Autodesk Fusion 360 part; units mm, degrees
note: some values were not read from the file. Chosen so that the rebuilt part matches the saved one: which bodies a step acts on; which sketch regions a step uses.
(part 5 of 6)
  line L2431 (-63.4833, -19.2831) -> (-62.2333, -17.118)
  line L2432 (-58.4101, -17.868) -> (-60.9101, -17.868)
  line L2433 (-67.2824, -20.0331) -> (-68.5324, -17.868)
  line L2434 (-88.7768, -22.1981) -> (-87.5268, -20.0331)
  line L2435 (-57.1601, -20.0331) -> (-58.4101, -17.868)
  line L2436 (-81.1546, -22.1981) -> (-78.6546, -22.1981)
  line L2437 (-98.899, -16.5315) -> (-97.649, -14.3664)
  line L2438 (-53.3611, -19.2831) -> (-52.1111, -17.118)
  line L2439 (-92.6, -17.118) -> (-93.85, -14.9529)
  line L2440 (-88.7768, -17.868) -> (-91.2768, -17.868)
  line L2441 (-91.2768, -17.868) -> (-92.5268, -20.0331)
  line L2442 (-62.2333, -17.118) -> (-63.4833, -14.9529)
  line L2443 (-7.799, -17.868) -> (-10.299, -17.868)
  line L2444 (-92.5268, -20.0331) -> (-91.2768, -22.1981)
  line L2445 (-78.6546, -22.1981) -> (-77.4046, -20.0331)
  line L2446 (-93.85, -14.9529) -> (-96.35, -14.9529)
  line L2447 (-96.35, -14.9529) -> (-97.6, -17.118)
  line L2448 (-82.4778, -17.118) -> (-83.7278, -14.9529)
  line L2449 (-73.6056, -19.2831) -> (-72.3556, -17.118)
  line L2450 (-6.5, -17.118) -> (-5.25, -19.2831)
  line L2451 (-50.7879, -22.1981) -> (-48.2879, -22.1981)
  line L2452 (-72.2824, -20.0331) -> (-71.0324, -22.1981)
  line L2453 (-101.399, -17.868) -> (-102.649, -20.0331)
  line L2454 (-58.4101, -22.1981) -> (-57.1601, -20.0331)
  line L2455 (-62.1601, -20.0331) -> (-60.9101, -22.1981)
  line L2456 (-47.0379, -20.0331) -> (-48.2879, -17.868)
  line L2457 (-98.899, -22.1981) -> (-97.649, -20.0331)
  line L2458 (-82.4046, -20.0331) -> (-81.1546, -22.1981)
  line L2459 (-5.25, -19.2831) -> (-2.75, -19.2831)
  line L2460 (-86.2278, -19.2831) -> (-83.7278, -19.2831)
  line L2461 (-55.8611, -14.9529) -> (-57.1111, -17.118)
  line L2462 (-55.8611, -19.2831) -> (-53.3611, -19.2831)
  line L2463 (-57.1111, -17.118) -> (-55.8611, -19.2831)
  line L2464 (-81.1546, -17.868) -> (-82.4046, -20.0331)
  line L2465 (-36.9157, -25.6997) -> (-38.1657, -23.5347)
  line L2466 (-52.0379, -25.6997) -> (-50.7879, -27.8648)
  line L2467 (-53.3611, -24.9497) -> (-52.1111, -22.7847)
  line L2468 (-50.7879, -27.8648) -> (-48.2879, -27.8648)
  line L2469 (-5.25, -20.6196) -> (-6.5, -22.7847)
  line L2470 (-28.0435, -27.8648) -> (-26.7935, -25.6997)
  line L2471 (-30.5435, -23.5347) -> (-31.7935, -25.6997)
  line L2472 (-38.1657, -23.5347) -> (-40.6657, -23.5347)
  line L2473 (-21.7444, -22.7847) -> (-22.9944, -20.6196)
  line L2474 (-68.5324, -17.868) -> (-71.0324, -17.868)
  line L2475 (-45.7389, -20.6196) -> (-46.9889, -22.7847)
  line L2476 (-71.0324, -17.868) -> (-72.2824, -20.0331)
  line L2477 (-22.9944, -24.9497) -> (-21.7444, -22.7847)
  line L2478 (-43.2389, -24.9497) -> (-41.9889, -22.7847)
  line L2479 (-36.8667, -22.7847) -> (-35.6167, -24.9497)
  line L2480 (-7.799, -27.8648) -> (-6.549, -25.6997)
  line L2481 (-40.6657, -23.5347) -> (-41.9157, -25.6997)
  line L2482 (-35.6167, -24.9497) -> (-33.1167, -24.9497)
  line L2483 (-22.9944, -20.6196) -> (-25.4944, -20.6196)
  line L2484 (-35.6167, -20.6196) -> (-36.8667, -22.7847)
  line L2485 (-48.2879, -22.1981) -> (-47.0379, -20.0331)
  line L2486 (-21.6713, -25.6997) -> (-20.4213, -27.8648)
  line L2487 (-38.1657, -27.8648) -> (-36.9157, -25.6997)
  line L2488 (-93.85, -19.2831) -> (-92.6, -17.118)
  line L2489 (-11.6222, -22.7847) -> (-12.8722, -20.6196)
  line L2490 (-20.4213, -23.5347) -> (-21.6713, -25.6997)
  line L2491 (-96.35, -19.2831) -> (-93.85, -19.2831)
  line L2492 (-5.25, -24.9497) -> (-2.75, -24.9497)
  line L2493 (-97.649, -20.0331) -> (-98.899, -17.868)
  line L2494 (-2.75, -24.9497) -> (-1.5, -22.7847)
  line L2495 (-16.6713, -25.6997) -> (-17.9213, -23.5347)
  line L2496 (-6.549, -25.6997) -> (-7.799, -23.5347)
  line L2497 (-41.9157, -25.6997) -> (-40.6657, -27.8648)
  line L2498 (-17.9213, -23.5347) -> (-20.4213, -23.5347)
  line L2499 (-31.8667, -22.7847) -> (-33.1167, -20.6196)
  line L2500 (-12.8722, -24.9497) -> (-11.6222, -22.7847)
  line L2501 (-17.9213, -27.8648) -> (-16.6713, -25.6997)
  line L2502 (-55.8611, -24.9497) -> (-53.3611, -24.9497)
  line L2503 (-6.5, -22.7847) -> (-5.25, -24.9497)
  line L2504 (-53.3611, -20.6196) -> (-55.8611, -20.6196)
  line L2505 (-33.1167, -24.9497) -> (-31.8667, -22.7847)
  line L2506 (-30.5435, -27.8648) -> (-28.0435, -27.8648)
  line L2507 (-31.7935, -25.6997) -> (-30.5435, -27.8648)
  line L2508 (-2.75, -20.6196) -> (-5.25, -20.6196)
  line L2509 (-45.7389, -24.9497) -> (-43.2389, -24.9497)
  line L2510 (-26.7935, -25.6997) -> (-28.0435, -23.5347)
  line L2511 (-11.549, -25.6997) -> (-10.299, -27.8648)
  line L2512 (-55.8611, -20.6196) -> (-57.1111, -22.7847)
  line L2513 (-41.9889, -22.7847) -> (-43.2389, -20.6196)
  line L2514 (-57.1111, -22.7847) -> (-55.8611, -24.9497)
  line L2515 (-77.3556, -17.118) -> (-76.1056, -19.2831)
  line L2516 (-1.5, -22.7847) -> (-2.75, -20.6196)
  line L2517 (-47.0379, -25.6997) -> (-48.2879, -23.5347)
  line L2518 (-12.8722, -20.6196) -> (-15.3722, -20.6196)
  line L2519 (-40.6657, -27.8648) -> (-38.1657, -27.8648)
  line L2520 (-20.4213, -27.8648) -> (-17.9213, -27.8648)
  line L2521 (-71.0324, -22.1981) -> (-68.5324, -22.1981)
  line L2522 (-87.4778, -17.118) -> (-86.2278, -19.2831)
  line L2523 (-48.2879, -23.5347) -> (-50.7879, -23.5347)
  line L2524 (-26.7444, -22.7847) -> (-25.4944, -24.9497)
  line L2525 (-65.9833, -19.2831) -> (-63.4833, -19.2831)
  line L2526 (-28.0435, -23.5347) -> (-30.5435, -23.5347)
  line L2527 (-43.2389, -20.6196) -> (-45.7389, -20.6196)
  line L2528 (-48.2879, -27.8648) -> (-47.0379, -25.6997)
  line L2529 (-2.75, -26.2863) -> (-5.25, -26.2863)
  line L2530 (-71.0324, -23.5347) -> (-72.2824, -25.6997)
  line L2531 (-68.5324, -27.8648) -> (-67.2824, -25.6997)
  line L2532 (-11.549, -31.3664) -> (-10.299, -33.5315)
  line L2533 (-91.2768, -27.8648) -> (-88.7768, -27.8648)
  line L2534 (-81.1546, -27.8648) -> (-78.6546, -27.8648)
  line L2535 (-93.85, -24.9497) -> (-92.6, -22.7847)
  line L2536 (-10.299, -23.5347) -> (-11.549, -25.6997)
  line L2537 (-15.3722, -24.9497) -> (-12.8722, -24.9497)
  line L2538 (-78.6546, -23.5347) -> (-81.1546, -23.5347)
  line L2539 (-60.9101, -23.5347) -> (-62.1601, -25.6997)
  line L2540 (-81.1546, -23.5347) -> (-82.4046, -25.6997)
  line L2541 (-65.9833, -20.6196) -> (-67.2333, -22.7847)
  line L2542 (-33.1167, -20.6196) -> (-35.6167, -20.6196)
  line L2543 (-58.4101, -23.5347) -> (-60.9101, -23.5347)
  line L2544 (-76.1056, -20.6196) -> (-77.3556, -22.7847)
  line L2545 (-25.4944, -24.9497) -> (-22.9944, -24.9497)
  line L2546 (-86.2278, -24.9497) -> (-83.7278, -24.9497)
  line L2547 (-97.6, -22.7847) -> (-96.35, -24.9497)
  line L2548 (-6.5, -28.4513) -> (-5.25, -30.6164)
  line L2549 (-63.4833, -20.6196) -> (-65.9833, -20.6196)
  line L2550 (-65.9833, -24.9497) -> (-63.4833, -24.9497)
  line L2551 (-88.7768, -27.8648) -> (-87.5268, -25.6997)
  line L2552 (-67.2824, -25.6997) -> (-68.5324, -23.5347)
  line L2553 (-2.75, -30.6164) -> (-1.5, -28.4513)
  line L2554 (-93.85, -20.6196) -> (-96.35, -20.6196)
  line L2555 (-98.899, -23.5347) -> (-101.399, -23.5347)
  line L2556 (-62.2333, -22.7847) -> (-63.4833, -20.6196)
  line L2557 (-92.6, -22.7847) -> (-93.85, -20.6196)
  line L2558 (-76.1056, -24.9497) -> (-73.6056, -24.9497)
  line L2559 (-96.35, -20.6196) -> (-97.6, -22.7847)
  line L2560 (-97.649, -25.6997) -> (-98.899, -23.5347)
  line L2561 (-7.799, -29.2013) -> (-10.299, -29.2013)
  line L2562 (-83.7278, -20.6196) -> (-86.2278, -20.6196)
  line L2563 (-73.6056, -20.6196) -> (-76.1056, -20.6196)
  line L2564 (-87.5268, -25.6997) -> (-88.7768, -23.5347)
  line L2565 (-83.7278, -24.9497) -> (-82.4778, -22.7847)
  line L2566 (-77.3556, -22.7847) -> (-76.1056, -24.9497)
  line L2567 (-88.7768, -23.5347) -> (-91.2768, -23.5347)
  line L2568 (-7.799, -23.5347) -> (-10.299, -23.5347)
  line L2569 (-15.3722, -20.6196) -> (-16.6222, -22.7847)
  line L2570 (-67.2333, -22.7847) -> (-65.9833, -24.9497)
  line L2571 (-1.5, -28.4513) -> (-2.75, -26.2863)
  line L2572 (-52.1111, -22.7847) -> (-53.3611, -20.6196)
  line L2573 (-25.4944, -20.6196) -> (-26.7444, -22.7847)
  line L2574 (-10.299, -29.2013) -> (-11.549, -31.3664)
  line L2575 (-101.399, -27.8648) -> (-98.899, -27.8648)
  line L2576 (-10.299, -33.5315) -> (-7.799, -33.5315)
  line L2577 (-72.3556, -22.7847) -> (-73.6056, -20.6196)
  line L2578 (-16.6222, -22.7847) -> (-15.3722, -24.9497)
  line L2579 (-92.5268, -25.6997) -> (-91.2768, -27.8648)
  line L2580 (-46.9889, -22.7847) -> (-45.7389, -24.9497)
  line L2581 (-10.299, -27.8648) -> (-7.799, -27.8648)
  line L2582 (-50.7879, -23.5347) -> (-52.0379, -25.6997)
  line L2583 (-58.4101, -27.8648) -> (-57.1601, -25.6997)
  line L2584 (-82.4046, -25.6997) -> (-81.1546, -27.8648)
  line L2585 (-72.2824, -25.6997) -> (-71.0324, -27.8648)
  line L2586 (-5.25, -30.6164) -> (-2.75, -30.6164)
  line L2587 (-87.4778, -22.7847) -> (-86.2278, -24.9497)
  line L2588 (-5.25, -26.2863) -> (-6.5, -28.4513)
  line L2589 (-62.1601, -25.6997) -> (-60.9101, -27.8648)
  line L2590 (-101.399, -23.5347) -> (-102.649, -25.6997)
  line L2591 (-102.649, -25.6997) -> (-101.399, -27.8648)
  line L2592 (-57.1601, -25.6997) -> (-58.4101, -23.5347)
  line L2593 (-30.5435, -33.5315) -> (-28.0435, -33.5315)
  line L2594 (-33.1167, -30.6164) -> (-31.8667, -28.4513)
  line L2595 (-50.7879, -29.2013) -> (-52.0379, -31.3664)
  line L2596 (-43.2389, -30.6164) -> (-41.9889, -28.4513)
  line L2597 (-91.2768, -23.5347) -> (-92.5268, -25.6997)
  line L2598 (-57.1111, -28.4513) -> (-55.8611, -30.6164)
  line L2599 (-20.4213, -33.5315) -> (-17.9213, -33.5315)
  line L2600 (-53.3611, -26.2863) -> (-55.8611, -26.2863)
  line L2601 (-26.7935, -31.3664) -> (-28.0435, -29.2013)
  line L2602 (-50.7879, -33.5315) -> (-48.2879, -33.5315)
  line L2603 (-71.0324, -27.8648) -> (-68.5324, -27.8648)
  line L2604 (-17.9213, -29.2013) -> (-20.4213, -29.2013)
  line L2605 (-26.7444, -28.4513) -> (-25.4944, -30.6164)
  line L2606 (-16.6713, -31.3664) -> (-17.9213, -29.2013)
  line L2607 (-77.4046, -25.6997) -> (-78.6546, -23.5347)
  line L2608 (-41.9157, -31.3664) -> (-40.6657, -33.5315)
  line L2609 (-41.9889, -28.4513) -> (-43.2389, -26.2863)
  line L2610 (-78.6546, -27.8648) -> (-77.4046, -25.6997)
  line L2611 (-86.2278, -20.6196) -> (-87.4778, -22.7847)
  line L2612 (-15.3722, -30.6164) -> (-12.8722, -30.6164)
  line L2613 (-63.4833, -24.9497) -> (-62.2333, -22.7847)
  line L2614 (-53.3611, -30.6164) -> (-52.1111, -28.4513)
  line L2615 (-40.6657, -33.5315) -> (-38.1657, -33.5315)
  line L2616 (-55.8611, -30.6164) -> (-53.3611, -30.6164)
  line L2617 (-16.6222, -28.4513) -> (-15.3722, -30.6164)
  line L2618 (-21.6713, -31.3664) -> (-20.4213, -33.5315)
  line L2619 (-15.3722, -26.2863) -> (-16.6222, -28.4513)
  line L2620 (-43.2389, -26.2863) -> (-45.7389, -26.2863)
  line L2621 (-11.6222, -28.4513) -> (-12.8722, -26.2863)
  line L2622 (-31.7935, -31.3664) -> (-30.5435, -33.5315)
  line L2623 (-28.0435, -29.2013) -> (-30.5435, -29.2013)
  line L2624 (-55.8611, -26.2863) -> (-57.1111, -28.4513)
  line L2625 (-38.1657, -33.5315) -> (-36.9157, -31.3664)
  line L2626 (-28.0435, -33.5315) -> (-26.7935, -31.3664)
  line L2627 (-48.2879, -29.2013) -> (-50.7879, -29.2013)
  line L2628 (-35.6167, -26.2863) -> (-36.8667, -28.4513)
  line L2629 (-98.899, -27.8648) -> (-97.649, -25.6997)
  line L2630 (-25.4944, -26.2863) -> (-26.7444, -28.4513)
  line L2631 (-52.1111, -28.4513) -> (-53.3611, -26.2863)
  line L2632 (-96.35, -24.9497) -> (-93.85, -24.9497)
  line L2633 (-20.4213, -29.2013) -> (-21.6713, -31.3664)
  line L2634 (-12.8722, -26.2863) -> (-15.3722, -26.2863)
  line L2635 (-58.4101, -29.2013) -> (-60.9101, -29.2013)
  line L2636 (-58.4101, -33.5315) -> (-57.1601, -31.3664)
  line L2637 (-52.0379, -31.3664) -> (-50.7879, -33.5315)
  line L2638 (-40.6657, -29.2013) -> (-41.9157, -31.3664)
  line L2639 (-82.4778, -22.7847) -> (-83.7278, -20.6196)
  line L2640 (-31.8667, -28.4513) -> (-33.1167, -26.2863)
  line L2641 (-47.0379, -31.3664) -> (-48.2879, -29.2013)
  line L2642 (-21.7444, -28.4513) -> (-22.9944, -26.2863)
  line L2643 (-60.9101, -27.8648) -> (-58.4101, -27.8648)
  line L2644 (-38.1657, -29.2013) -> (-40.6657, -29.2013)
  line L2645 (-48.2879, -33.5315) -> (-47.0379, -31.3664)
  line L2646 (-36.9157, -31.3664) -> (-38.1657, -29.2013)
  line L2647 (-46.9889, -28.4513) -> (-45.7389, -30.6164)
  line L2648 (-6.549, -31.3664) -> (-7.799, -29.2013)
  line L2649 (-33.1167, -26.2863) -> (-35.6167, -26.2863)
  line L2650 (-45.7389, -26.2863) -> (-46.9889, -28.4513)
  line L2651 (-73.6056, -24.9497) -> (-72.3556, -22.7847)
  line L2652 (-36.8667, -28.4513) -> (-35.6167, -30.6164)
  line L2653 (-17.9213, -33.5315) -> (-16.6713, -31.3664)
  line L2654 (-62.1601, -31.3664) -> (-60.9101, -33.5315)
  line L2655 (-60.9101, -29.2013) -> (-62.1601, -31.3664)
  line L2656 (-68.5324, -23.5347) -> (-71.0324, -23.5347)
  line L2657 (-2.75, -36.2831) -> (-1.5, -34.118)
  line L2658 (-7.799, -34.868) -> (-10.299, -34.868)
  line L2659 (-11.6222, -34.118) -> (-12.8722, -31.9529)
  line L2660 (-83.7278, -26.2863) -> (-86.2278, -26.2863)
  line L2661 (-30.5435, -29.2013) -> (-31.7935, -31.3664)
  line L2662 (-98.899, -33.5315) -> (-97.649, -31.3664)
  line L2663 (-1.5, -34.118) -> (-2.75, -31.9529)
  line L2664 (-81.1546, -29.2013) -> (-82.4046, -31.3664)
  line L2665 (-35.6167, -30.6164) -> (-33.1167, -30.6164)
  line L2666 (-63.4833, -30.6164) -> (-62.2333, -28.4513)
  line L2667 (-67.2824, -31.3664) -> (-68.5324, -29.2013)
  line L2668 (-45.7389, -30.6164) -> (-43.2389, -30.6164)
  line L2669 (-78.6546, -29.2013) -> (-81.1546, -29.2013)
  line L2670 (-97.6, -28.4513) -> (-96.35, -30.6164)
  line L2671 (-25.4944, -30.6164) -> (-22.9944, -30.6164)
  line L2672 (-12.8722, -31.9529) -> (-15.3722, -31.9529)
  line L2673 (-93.85, -26.2863) -> (-96.35, -26.2863)
  line L2674 (-63.4833, -26.2863) -> (-65.9833, -26.2863)
  line L2675 (-87.5268, -31.3664) -> (-88.7768, -29.2013)
  line L2676 (-7.799, -33.5315) -> (-6.549, -31.3664)
  line L2677 (-91.2768, -29.2013) -> (-92.5268, -31.3664)
  line L2678 (-73.6056, -26.2863) -> (-76.1056, -26.2863)
  line L2679 (-102.649, -31.3664) -> (-101.399, -33.5315)
  line L2680 (-7.799, -39.1981) -> (-6.549, -37.0331)
  line L2681 (-11.549, -37.0331) -> (-10.299, -39.1981)
  line L2682 (-73.6056, -30.6164) -> (-72.3556, -28.4513)
  line L2683 (-57.1601, -31.3664) -> (-58.4101, -29.2013)
  line L2684 (-88.7768, -29.2013) -> (-91.2768, -29.2013)
  line L2685 (-22.9944, -30.6164) -> (-21.7444, -28.4513)
  line L2686 (-86.2278, -26.2863) -> (-87.4778, -28.4513)
  line L2687 (-101.399, -33.5315) -> (-98.899, -33.5315)
  line L2688 (-82.4046, -31.3664) -> (-81.1546, -33.5315)
  line L2689 (-92.6, -28.4513) -> (-93.85, -26.2863)
  line L2690 (-67.2333, -28.4513) -> (-65.9833, -30.6164)
  line L2691 (-76.1056, -26.2863) -> (-77.3556, -28.4513)
  line L2692 (-5.25, -31.9529) -> (-6.5, -34.118)
  line L2693 (-72.2824, -31.3664) -> (-71.0324, -33.5315)
  line L2694 (-96.35, -30.6164) -> (-93.85, -30.6164)
  line L2695 (-97.649, -31.3664) -> (-98.899, -29.2013)
  line L2696 (-101.399, -29.2013) -> (-102.649, -31.3664)
  line L2697 (-68.5324, -33.5315) -> (-67.2824, -31.3664)
  line L2698 (-77.3556, -28.4513) -> (-76.1056, -30.6164)
  line L2699 (-91.2768, -33.5315) -> (-88.7768, -33.5315)
  line L2700 (-10.299, -39.1981) -> (-7.799, -39.1981)
  line L2701 (-96.35, -26.2863) -> (-97.6, -28.4513)
  line L2702 (-62.2333, -28.4513) -> (-63.4833, -26.2863)
  line L2703 (-12.8722, -30.6164) -> (-11.6222, -28.4513)
  line L2704 (-60.9101, -33.5315) -> (-58.4101, -33.5315)
  line L2705 (-22.9944, -26.2863) -> (-25.4944, -26.2863)
  line L2706 (-12.8722, -36.2831) -> (-11.6222, -34.118)
  line L2707 (-6.549, -37.0331) -> (-7.799, -34.868)
  line L2708 (-93.85, -30.6164) -> (-92.6, -28.4513)
  line L2709 (-76.1056, -30.6164) -> (-73.6056, -30.6164)
  line L2710 (-68.5324, -29.2013) -> (-71.0324, -29.2013)
  line L2711 (-82.4778, -28.4513) -> (-83.7278, -26.2863)
  line L2712 (-98.899, -29.2013) -> (-101.399, -29.2013)
  line L2713 (-71.0324, -33.5315) -> (-68.5324, -33.5315)
  line L2714 (-72.3556, -28.4513) -> (-73.6056, -26.2863)
  line L2715 (-65.9833, -30.6164) -> (-63.4833, -30.6164)
  line L2716 (-71.0324, -29.2013) -> (-72.2824, -31.3664)
  line L2717 (-10.299, -34.868) -> (-11.549, -37.0331)
  line L2718 (-5.25, -36.2831) -> (-2.75, -36.2831)
  line L2719 (-6.5, -34.118) -> (-5.25, -36.2831)
  line L2720 (-86.2278, -30.6164) -> (-83.7278, -30.6164)
  line L2721 (-30.5435, -34.868) -> (-31.7935, -37.0331)
  line L2722 (-38.1657, -34.868) -> (-40.6657, -34.868)
  line L2723 (-53.3611, -31.9529) -> (-55.8611, -31.9529)
  line L2724 (-58.4101, -39.1981) -> (-57.1601, -37.0331)
  line L2725 (-47.0379, -37.0331) -> (-48.2879, -34.868)
  line L2726 (-31.7935, -37.0331) -> (-30.5435, -39.1981)
  line L2727 (-68.5324, -34.868) -> (-71.0324, -34.868)
  line L2728 (-71.0324, -34.868) -> (-72.2824, -37.0331)
  line L2729 (-46.9889, -34.118) -> (-45.7389, -36.2831)
  line L2730 (-71.0324, -39.1981) -> (-68.5324, -39.1981)
  line L2731 (-17.9213, -34.868) -> (-20.4213, -34.868)
  line L2732 (-41.9889, -34.118) -> (-43.2389, -31.9529)
  line L2733 (-52.0379, -37.0331) -> (-50.7879, -39.1981)
  line L2734 (-17.9213, -39.1981) -> (-16.6713, -37.0331)
  line L2735 (-92.5268, -31.3664) -> (-91.2768, -33.5315)
  line L2736 (-22.9944, -36.2831) -> (-21.7444, -34.118)
  line L2737 (-31.8667, -34.118) -> (-33.1167, -31.9529)
  line L2738 (-41.9157, -37.0331) -> (-40.6657, -39.1981)
  line L2739 (-25.4944, -36.2831) -> (-22.9944, -36.2831)
  line L2740 (-20.4213, -39.1981) -> (-17.9213, -39.1981)
  line L2741 (-65.9833, -36.2831) -> (-63.4833, -36.2831)
  line L2742 (-58.4101, -34.868) -> (-60.9101, -34.868)
  line L2743 (-15.3722, -36.2831) -> (-12.8722, -36.2831)
  line L2744 (-88.7768, -33.5315) -> (-87.5268, -31.3664)
  line L2745 (-30.5435, -39.1981) -> (-28.0435, -39.1981)
  line L2746 (-60.9101, -34.868) -> (-62.1601, -37.0331)
  line L2747 (-25.4944, -31.9529) -> (-26.7444, -34.118)
  line L2748 (-21.6713, -37.0331) -> (-20.4213, -39.1981)
  line L2749 (-40.6657, -39.1981) -> (-38.1657, -39.1981)
  line L2750 (-38.1657, -39.1981) -> (-36.9157, -37.0331)
  line L2751 (-40.6657, -34.868) -> (-41.9157, -37.0331)
  line L2752 (-48.2879, -34.868) -> (-50.7879, -34.868)
  line L2753 (-57.1111, -34.118) -> (-55.8611, -36.2831)
  line L2754 (-52.1111, -34.118) -> (-53.3611, -31.9529)
  line L2755 (-60.9101, -39.1981) -> (-58.4101, -39.1981)
  line L2756 (-28.0435, -39.1981) -> (-26.7935, -37.0331)
  line L2757 (-83.7278, -30.6164) -> (-82.4778, -28.4513)
  line L2758 (-2.75, -31.9529) -> (-5.25, -31.9529)
  line L2759 (-16.6222, -34.118) -> (-15.3722, -36.2831)
  line L2760 (-77.4046, -31.3664) -> (-78.6546, -29.2013)
  line L2761 (-22.9944, -31.9529) -> (-25.4944, -31.9529)
  line L2762 (-26.7444, -34.118) -> (-25.4944, -36.2831)
  line L2763 (-35.6167, -36.2831) -> (-33.1167, -36.2831)
  line L2764 (-65.9833, -31.9529) -> (-67.2333, -34.118)
  line L2765 (-72.2824, -37.0331) -> (-71.0324, -39.1981)
  line L2766 (-16.6713, -37.0331) -> (-17.9213, -34.868)
  line L2767 (-65.9833, -26.2863) -> (-67.2333, -28.4513)
  line L2768 (-62.2333, -34.118) -> (-63.4833, -31.9529)
  line L2769 (-45.7389, -31.9529) -> (-46.9889, -34.118)
  line L2770 (-36.8667, -34.118) -> (-35.6167, -36.2831)
  line L2771 (-62.1601, -37.0331) -> (-60.9101, -39.1981)
  line L2772 (-33.1167, -36.2831) -> (-31.8667, -34.118)
  line L2773 (-50.7879, -34.868) -> (-52.0379, -37.0331)
  line L2774 (-63.4833, -31.9529) -> (-65.9833, -31.9529)
  line L2775 (-43.2389, -31.9529) -> (-45.7389, -31.9529)
  line L2776 (-78.6546, -33.5315) -> (-77.4046, -31.3664)
  line L2777 (-87.4778, -28.4513) -> (-86.2278, -30.6164)
  line L2778 (-63.4833, -36.2831) -> (-62.2333, -34.118)
  line L2779 (-55.8611, -31.9529) -> (-57.1111, -34.118)
  line L2780 (-81.1546, -33.5315) -> (-78.6546, -33.5315)
  line L2781 (-20.4213, -34.868) -> (-21.6713, -37.0331)
  line L2782 (-15.3722, -31.9529) -> (-16.6222, -34.118)
  line L2783 (-33.1167, -31.9529) -> (-35.6167, -31.9529)
  line L2784 (-53.3611, -36.2831) -> (-52.1111, -34.118)
  line L2785 (-5.25, -37.6196) -> (-6.5, -39.7847)
  line L2786 (-21.7444, -34.118) -> (-22.9944, -31.9529)
  line L2787 (-97.6, -34.118) -> (-96.35, -36.2831)
  line L2788 (-36.9157, -37.0331) -> (-38.1657, -34.868)
  line L2789 (-11.549, -42.6997) -> (-10.299, -44.8648)
  line L2790 (-50.7879, -39.1981) -> (-48.2879, -39.1981)
  line L2791 (-15.3722, -41.9497) -> (-12.8722, -41.9497)
  line L2792 (-82.4046, -37.0331) -> (-81.1546, -39.1981)
  line L2793 (-28.0435, -34.868) -> (-30.5435, -34.868)
  line L2794 (-21.6713, -42.6997) -> (-20.4213, -44.8648)
  line L2795 (-15.3722, -37.6196) -> (-16.6222, -39.7847)
  line L2796 (-82.4778, -34.118) -> (-83.7278, -31.9529)
  line L2797 (-92.5268, -37.0331) -> (-91.2768, -39.1981)
  line L2798 (-72.3556, -34.118) -> (-73.6056, -31.9529)
  line L2799 (-11.6222, -39.7847) -> (-12.8722, -37.6196)
  line L2800 (-77.4046, -37.0331) -> (-78.6546, -34.868)
  line L2801 (-26.7935, -37.0331) -> (-28.0435, -34.868)
  line L2802 (-10.299, -44.8648) -> (-7.799, -44.8648)
  line L2803 (-68.5324, -39.1981) -> (-67.2824, -37.0331)
  line L2804 (-86.2278, -36.2831) -> (-83.7278, -36.2831)
  line L2805 (-81.1546, -39.1981) -> (-78.6546, -39.1981)
  line L2806 (-87.5268, -37.0331) -> (-88.7768, -34.868)
  line L2807 (-96.35, -31.9529) -> (-97.6, -34.118)
  line L2808 (-26.7444, -39.7847) -> (-25.4944, -41.9497)
  line L2809 (-102.649, -37.0331) -> (-101.399, -39.1981)
  line L2810 (-12.8722, -37.6196) -> (-15.3722, -37.6196)
  line L2811 (-12.8722, -41.9497) -> (-11.6222, -39.7847)
  line L2812 (-57.1601, -37.0331) -> (-58.4101, -34.868)
  line L2813 (-25.4944, -41.9497) -> (-22.9944, -41.9497)
  line L2814 (-76.1056, -31.9529) -> (-77.3556, -34.118)
  line L2815 (-1.5, -39.7847) -> (-2.75, -37.6196)
  line L2816 (-67.2824, -37.0331) -> (-68.5324, -34.868)
  line L2817 (-91.2768, -39.1981) -> (-88.7768, -39.1981)
  line L2818 (-7.799, -40.5347) -> (-10.299, -40.5347)
  line L2819 (-55.8611, -36.2831) -> (-53.3611, -36.2831)
  line L2820 (-87.4778, -34.118) -> (-86.2278, -36.2831)
  line L2821 (-96.35, -36.2831) -> (-93.85, -36.2831)
  line L2822 (-7.799, -44.8648) -> (-6.549, -42.6997)
  line L2823 (-83.7278, -31.9529) -> (-86.2278, -31.9529)
  line L2824 (-43.2389, -36.2831) -> (-41.9889, -34.118)
  line L2825 (-35.6167, -31.9529) -> (-36.8667, -34.118)
  line L2826 (-97.649, -37.0331) -> (-98.899, -34.868)
  line L2827 (-67.2333, -34.118) -> (-65.9833, -36.2831)
  line L2828 (-98.899, -34.868) -> (-101.399, -34.868)
  line L2829 (-81.1546, -34.868) -> (-82.4046, -37.0331)
  line L2830 (-101.399, -34.868) -> (-102.649, -37.0331)
  line L2831 (-20.4213, -44.8648) -> (-17.9213, -44.8648)
  line L2832 (-48.2879, -39.1981) -> (-47.0379, -37.0331)
  line L2833 (-78.6546, -39.1981) -> (-77.4046, -37.0331)
  line L2834 (-2.75, -41.9497) -> (-1.5, -39.7847)
  line L2835 (-92.6, -34.118) -> (-93.85, -31.9529)
  line L2836 (-93.85, -31.9529) -> (-96.35, -31.9529)
  line L2837 (-78.6546, -34.868) -> (-81.1546, -34.868)
  line L2838 (-45.7389, -36.2831) -> (-43.2389, -36.2831)
  line L2839 (-10.299, -40.5347) -> (-11.549, -42.6997)
  line L2840 (-2.75, -37.6196) -> (-5.25, -37.6196)
  line L2841 (-20.4213, -40.5347) -> (-21.6713, -42.6997)
  line L2842 (-73.6056, -31.9529) -> (-76.1056, -31.9529)
  line L2843 (-6.5, -39.7847) -> (-5.25, -41.9497)
  line L2844 (-73.6056, -36.2831) -> (-72.3556, -34.118)
  line L2845 (-16.6713, -42.6997) -> (-17.9213, -40.5347)
  line L2846 (-76.1056, -36.2831) -> (-73.6056, -36.2831)
  line L2847 (-91.2768, -34.868) -> (-92.5268, -37.0331)
  line L2848 (-17.9213, -40.5347) -> (-20.4213, -40.5347)
  line L2849 (-53.3611, -41.9497) -> (-52.1111, -39.7847)
  line L2850 (-58.4101, -44.8648) -> (-57.1601, -42.6997)
  line L2851 (-31.7935, -42.6997) -> (-30.5435, -44.8648)
  line L2852 (-62.1601, -42.6997) -> (-60.9101, -44.8648)
  line L2853 (-67.2333, -39.7847) -> (-65.9833, -41.9497)
  line L2854 (-22.9944, -37.6196) -> (-25.4944, -37.6196)
  line L2855 (-46.9889, -39.7847) -> (-45.7389, -41.9497)
  line L2856 (-45.7389, -41.9497) -> (-43.2389, -41.9497)
  line L2857 (-40.6657, -44.8648) -> (-38.1657, -44.8648)
  line L2858 (-77.3556, -34.118) -> (-76.1056, -36.2831)
  line L2859 (-30.5435, -40.5347) -> (-31.7935, -42.6997)
  line L2860 (-16.6222, -39.7847) -> (-15.3722, -41.9497)
  line L2861 (-28.0435, -44.8648) -> (-26.7935, -42.6997)
  line L2862 (-28.0435, -40.5347) -> (-30.5435, -40.5347)
  line L2863 (-36.8667, -39.7847) -> (-35.6167, -41.9497)
  line L2864 (-45.7389, -37.6196) -> (-46.9889, -39.7847)
  line L2865 (-26.7935, -42.6997) -> (-28.0435, -40.5347)
  line L2866 (-31.8667, -39.7847) -> (-33.1167, -37.6196)
  line L2867 (-77.3556, -39.7847) -> (-76.1056, -41.9497)
  line L2868 (-41.9157, -42.6997) -> (-40.6657, -44.8648)
  line L2869 (-101.399, -39.1981) -> (-98.899, -39.1981)
  line L2870 (-67.2824, -42.6997) -> (-68.5324, -40.5347)
  line L2871 (-33.1167, -37.6196) -> (-35.6167, -37.6196)
  line L2872 (-98.899, -39.1981) -> (-97.649, -37.0331)
  line L2873 (-73.6056, -41.9497) -> (-72.3556, -39.7847)
  line L2874 (-22.9944, -41.9497) -> (-21.7444, -39.7847)
  line L2875 (-17.9213, -44.8648) -> (-16.6713, -42.6997)
  line L2876 (-86.2278, -31.9529) -> (-87.4778, -34.118)
  line L2877 (-5.25, -41.9497) -> (-2.75, -41.9497)
  line L2878 (-43.2389, -37.6196) -> (-45.7389, -37.6196)
  line L2879 (-60.9101, -40.5347) -> (-62.1601, -42.6997)
  line L2880 (-63.4833, -37.6196) -> (-65.9833, -37.6196)
  line L2881 (-76.1056, -41.9497) -> (-73.6056, -41.9497)
  line L2882 (-76.1056, -37.6196) -> (-77.3556, -39.7847)
  line L2883 (-48.2879, -40.5347) -> (-50.7879, -40.5347)
  line L2884 (-55.8611, -37.6196) -> (-57.1111, -39.7847)
  line L2885 (-52.0379, -42.6997) -> (-50.7879, -44.8648)
  line L2886 (-30.5435, -44.8648) -> (-28.0435, -44.8648)
  line L2887 (-83.7278, -36.2831) -> (-82.4778, -34.118)
  line L2888 (-43.2389, -41.9497) -> (-41.9889, -39.7847)
  line L2889 (-88.7768, -39.1981) -> (-87.5268, -37.0331)
  line L2890 (-73.6056, -37.6196) -> (-76.1056, -37.6196)
  line L2891 (-62.2333, -39.7847) -> (-63.4833, -37.6196)
  line L2892 (-57.1601, -42.6997) -> (-58.4101, -40.5347)
  line L2893 (-40.6657, -40.5347) -> (-41.9157, -42.6997)
  line L2894 (-41.9889, -39.7847) -> (-43.2389, -37.6196)
  line L2895 (-58.4101, -40.5347) -> (-60.9101, -40.5347)
  line L2896 (-47.0379, -42.6997) -> (-48.2879, -40.5347)
  line L2897 (-52.1111, -39.7847) -> (-53.3611, -37.6196)
  line L2898 (-65.9833, -41.9497) -> (-63.4833, -41.9497)
  line L2899 (-68.5324, -44.8648) -> (-67.2824, -42.6997)
  line L2900 (-55.8611, -41.9497) -> (-53.3611, -41.9497)
  line L2901 (-72.2824, -42.6997) -> (-71.0324, -44.8648)
  line L2902 (-35.6167, -41.9497) -> (-33.1167, -41.9497)
  line L2903 (-36.9157, -42.6997) -> (-38.1657, -40.5347)
  line L2904 (-72.3556, -39.7847) -> (-73.6056, -37.6196)
  line L2905 (-88.7768, -34.868) -> (-91.2768, -34.868)
  line L2906 (-93.85, -36.2831) -> (-92.6, -34.118)
  line L2907 (-21.7444, -39.7847) -> (-22.9944, -37.6196)
  line L2908 (-65.9833, -37.6196) -> (-67.2333, -39.7847)
  line L2909 (-6.549, -42.6997) -> (-7.799, -40.5347)
  line L2910 (-53.3611, -37.6196) -> (-55.8611, -37.6196)
  line L2911 (-25.4944, -37.6196) -> (-26.7444, -39.7847)
  line L2912 (-50.7879, -44.8648) -> (-48.2879, -44.8648)
  line L2913 (-25.4944, -43.2863) -> (-26.7444, -45.4513)
  line L2914 (-28.0435, -46.2013) -> (-30.5435, -46.2013)
  line L2915 (-31.7935, -48.3664) -> (-30.5435, -50.5315)
  line L2916 (-6.5, -45.4513) -> (-5.25, -47.6164)
  line L2917 (-21.7444, -45.4513) -> (-22.9944, -43.2863)
  line L2918 (-11.549, -48.3664) -> (-10.299, -50.5315)
  line L2919 (-97.6, -39.7847) -> (-96.35, -41.9497)
  line L2920 (-5.25, -47.6164) -> (-2.75, -47.6164)
  line L2921 (-96.35, -37.6196) -> (-97.6, -39.7847)
  line L2922 (-63.4833, -41.9497) -> (-62.2333, -39.7847)
  line L2923 (-87.5268, -42.6997) -> (-88.7768, -40.5347)
  line L2924 (-50.7879, -40.5347) -> (-52.0379, -42.6997)
  line L2925 (-98.899, -40.5347) -> (-101.399, -40.5347)
  line L2926 (-88.7768, -40.5347) -> (-91.2768, -40.5347)
  line L2927 (-81.1546, -40.5347) -> (-82.4046, -42.6997)
  line L2928 (-38.1657, -44.8648) -> (-36.9157, -42.6997)
  line L2929 (-82.4778, -39.7847) -> (-83.7278, -37.6196)
  line L2930 (-87.4778, -39.7847) -> (-86.2278, -41.9497)
  line L2931 (-83.7278, -41.9497) -> (-82.4778, -39.7847)
  line L2932 (-86.2278, -37.6196) -> (-87.4778, -39.7847)
  line L2933 (-68.5324, -40.5347) -> (-71.0324, -40.5347)
  line L2934 (-30.5435, -46.2013) -> (-31.7935, -48.3664)
  line L2935 (-30.5435, -50.5315) -> (-28.0435, -50.5315)
  line L2936 (-91.2768, -40.5347) -> (-92.5268, -42.6997)
  line L2937 (-12.8722, -47.6164) -> (-11.6222, -45.4513)
  line L2938 (-102.649, -42.6997) -> (-101.399, -44.8648)
  line L2939 (-20.4213, -46.2013) -> (-21.6713, -48.3664)
  line L2940 (-60.9101, -44.8648) -> (-58.4101, -44.8648)
  line L2941 (-7.799, -50.5315) -> (-6.549, -48.3664)
  line L2942 (-21.6713, -48.3664) -> (-20.4213, -50.5315)
  line L2943 (-2.75, -43.2863) -> (-5.25, -43.2863)
  line L2944 (-17.9213, -50.5315) -> (-16.6713, -48.3664)
  line L2945 (-20.4213, -50.5315) -> (-17.9213, -50.5315)
  line L2946 (-71.0324, -40.5347) -> (-72.2824, -42.6997)
  line L2947 (-15.3722, -43.2863) -> (-16.6222, -45.4513)
  line L2948 (-101.399, -40.5347) -> (-102.649, -42.6997)
  line L2949 (-86.2278, -41.9497) -> (-83.7278, -41.9497)
  line L2950 (-7.799, -46.2013) -> (-10.299, -46.2013)
  line L2951 (-6.549, -48.3664) -> (-7.799, -46.2013)
  line L2952 (-83.7278, -37.6196) -> (-86.2278, -37.6196)
  line L2953 (-10.299, -50.5315) -> (-7.799, -50.5315)
  line L2954 (-22.9944, -43.2863) -> (-25.4944, -43.2863)
  line L2955 (-93.85, -41.9497) -> (-92.6, -39.7847)
  line L2956 (-91.2768, -44.8648) -> (-88.7768, -44.8648)
  line L2957 (-26.7444, -45.4513) -> (-25.4944, -47.6164)
  line L2958 (-11.6222, -45.4513) -> (-12.8722, -43.2863)
  line L2959 (-33.1167, -41.9497) -> (-31.8667, -39.7847)
  line L2960 (-92.5268, -42.6997) -> (-91.2768, -44.8648)
  line L2961 (-38.1657, -40.5347) -> (-40.6657, -40.5347)
  line L2962 (-2.75, -47.6164) -> (-1.5, -45.4513)
  line L2963 (-22.9944, -47.6164) -> (-21.7444, -45.4513)
  line L2964 (-82.4046, -42.6997) -> (-81.1546, -44.8648)
  line L2965 (-93.85, -37.6196) -> (-96.35, -37.6196)
  line L2966 (-92.6, -39.7847) -> (-93.85, -37.6196)
  line L2967 (-81.1546, -44.8648) -> (-78.6546, -44.8648)
  line L2968 (-16.6713, -48.3664) -> (-17.9213, -46.2013)
  line L2969 (-35.6167, -37.6196) -> (-36.8667, -39.7847)
  line L2970 (-71.0324, -44.8648) -> (-68.5324, -44.8648)
  line L2971 (-98.899, -44.8648) -> (-97.649, -42.6997)
  line L2972 (-12.8722, -43.2863) -> (-15.3722, -43.2863)
  line L2973 (-48.2879, -44.8648) -> (-47.0379, -42.6997)
  line L2974 (-25.4944, -47.6164) -> (-22.9944, -47.6164)
  line L2975 (-78.6546, -40.5347) -> (-81.1546, -40.5347)
  line L2976 (-57.1111, -39.7847) -> (-55.8611, -41.9497)
  line L2977 (-68.5324, -46.2013) -> (-71.0324, -46.2013)
  line L2978 (-33.1167, -43.2863) -> (-35.6167, -43.2863)
  line L2979 (-40.6657, -46.2013) -> (-41.9157, -48.3664)
  line L2980 (-41.9889, -45.4513) -> (-43.2389, -43.2863)
  line L2981 (-78.6546, -44.8648) -> (-77.4046, -42.6997)
  line L2982 (-35.6167, -47.6164) -> (-33.1167, -47.6164)
  line L2983 (-68.5324, -50.5315) -> (-67.2824, -48.3664)
  line L2984 (-88.7768, -44.8648) -> (-87.5268, -42.6997)
  line L2985 (-48.2879, -46.2013) -> (-50.7879, -46.2013)
  line L2986 (-72.2824, -48.3664) -> (-71.0324, -50.5315)
  line L2987 (-10.299, -46.2013) -> (-11.549, -48.3664)
  line L2988 (-47.0379, -48.3664) -> (-48.2879, -46.2013)
  line L2989 (-53.3611, -47.6164) -> (-52.1111, -45.4513)
  line L2990 (-57.1111, -45.4513) -> (-55.8611, -47.6164)
  line L2991 (-17.9213, -46.2013) -> (-20.4213, -46.2013)
  line L2992 (-15.3722, -47.6164) -> (-12.8722, -47.6164)
  line L2993 (-65.9833, -47.6164) -> (-63.4833, -47.6164)
  line L2994 (-96.35, -41.9497) -> (-93.85, -41.9497)
  line L2995 (-97.649, -42.6997) -> (-98.899, -40.5347)
  line L2996 (-67.2824, -48.3664) -> (-68.5324, -46.2013)
  line L2997 (-67.2333, -45.4513) -> (-65.9833, -47.6164)
  line L2998 (-76.1056, -43.2863) -> (-77.3556, -45.4513)
  line L2999 (-63.4833, -43.2863) -> (-65.9833, -43.2863)
  line L3000 (-41.9157, -48.3664) -> (-40.6657, -50.5315)
  line L3001 (-43.2389, -43.2863) -> (-45.7389, -43.2863)
  line L3002 (-38.1657, -50.5315) -> (-36.9157, -48.3664)
  line L3003 (-5.25, -43.2863) -> (-6.5, -45.4513)
  line L3004 (-60.9101, -46.2013) -> (-62.1601, -48.3664)
  line L3005 (-52.0379, -48.3664) -> (-50.7879, -50.5315)
  line L3006 (-78.6546, -46.2013) -> (-81.1546, -46.2013)
  line L3007 (-77.3556, -45.4513) -> (-76.1056, -47.6164)
  line L3008 (-45.7389, -47.6164) -> (-43.2389, -47.6164)
  line L3009 (-65.9833, -43.2863) -> (-67.2333, -45.4513)
  line L3010 (-63.4833, -47.6164) -> (-62.2333, -45.4513)
  line L3011 (-71.0324, -46.2013) -> (-72.2824, -48.3664)
  line L3012 (-48.2879, -50.5315) -> (-47.0379, -48.3664)
  line L3013 (-1.5, -45.4513) -> (-2.75, -43.2863)
  line L3014 (-62.2333, -45.4513) -> (-63.4833, -43.2863)
  line L3015 (-36.8667, -45.4513) -> (-35.6167, -47.6164)
  line L3016 (-101.399, -44.8648) -> (-98.899, -44.8648)
  line L3017 (-52.1111, -45.4513) -> (-53.3611, -43.2863)
  line L3018 (-31.8667, -45.4513) -> (-33.1167, -43.2863)
  line L3019 (-73.6056, -47.6164) -> (-72.3556, -45.4513)
  line L3020 (-45.7389, -43.2863) -> (-46.9889, -45.4513)
  line L3021 (-40.6657, -50.5315) -> (-38.1657, -50.5315)
  line L3022 (-71.0324, -50.5315) -> (-68.5324, -50.5315)
  line L3023 (-62.1601, -48.3664) -> (-60.9101, -50.5315)
  line L3024 (-36.9157, -48.3664) -> (-38.1657, -46.2013)
  line L3025 (-28.0435, -50.5315) -> (-26.7935, -48.3664)
  line L3026 (-16.6222, -45.4513) -> (-15.3722, -47.6164)
  line L3027 (-77.4046, -42.6997) -> (-78.6546, -40.5347)
  line L3028 (-58.4101, -50.5315) -> (-57.1601, -48.3664)
  line L3029 (-35.6167, -43.2863) -> (-36.8667, -45.4513)
  line L3030 (-57.1601, -48.3664) -> (-58.4101, -46.2013)
  line L3031 (-73.6056, -43.2863) -> (-76.1056, -43.2863)
  line L3032 (-76.1056, -47.6164) -> (-73.6056, -47.6164)
  line L3033 (-58.4101, -46.2013) -> (-60.9101, -46.2013)
  line L3034 (-72.3556, -45.4513) -> (-73.6056, -43.2863)
  line L3035 (-55.8611, -43.2863) -> (-57.1111, -45.4513)
  line L3036 (-60.9101, -50.5315) -> (-58.4101, -50.5315)
  line L3037 (-50.7879, -46.2013) -> (-52.0379, -48.3664)
  line L3038 (-55.8611, -47.6164) -> (-53.3611, -47.6164)
  line L3039 (-53.3611, -43.2863) -> (-55.8611, -43.2863)
  line L3040 (-50.7879, -50.5315) -> (-48.2879, -50.5315)
  line L3041 (-12.8722, -53.2831) -> (-11.6222, -51.118)
  line L3042 (-96.35, -43.2863) -> (-97.6, -45.4513)
  line L3043 (-28.0435, -51.868) -> (-30.5435, -51.868)
  line L3044 (-30.5435, -56.1981) -> (-28.0435, -56.1981)
  line L3045 (-5.25, -53.2831) -> (-2.75, -53.2831)
  line L3046 (-6.549, -54.0331) -> (-7.799, -51.868)
  line L3047 (-25.4944, -48.9529) -> (-26.7444, -51.118)
  line L3048 (-36.8667, -51.118) -> (-35.6167, -53.2831)
  line L3049 (-97.649, -48.3664) -> (-98.899, -46.2013)
  line L3050 (-10.299, -51.868) -> (-11.549, -54.0331)
  line L3051 (-20.4213, -56.1981) -> (-17.9213, -56.1981)
  line L3052 (-10.299, -56.1981) -> (-7.799, -56.1981)
  line L3053 (-35.6167, -53.2831) -> (-33.1167, -53.2831)
  line L3054 (-101.399, -46.2013) -> (-102.649, -48.3664)
  line L3055 (-81.1546, -46.2013) -> (-82.4046, -48.3664)
  line L3056 (-38.1657, -46.2013) -> (-40.6657, -46.2013)
  line L3057 (-33.1167, -53.2831) -> (-31.8667, -51.118)
  line L3058 (-92.6, -45.4513) -> (-93.85, -43.2863)
  line L3059 (-20.4213, -51.868) -> (-21.6713, -54.0331)
  line L3060 (-31.8667, -51.118) -> (-33.1167, -48.9529)
  line L3061 (-16.6713, -54.0331) -> (-17.9213, -51.868)
  line L3062 (-17.9213, -56.1981) -> (-16.6713, -54.0331)
  line L3063 (-87.4778, -45.4513) -> (-86.2278, -47.6164)
  line L3064 (-43.2389, -47.6164) -> (-41.9889, -45.4513)
  line L3065 (-17.9213, -51.868) -> (-20.4213, -51.868)
  line L3066 (-86.2278, -43.2863) -> (-87.4778, -45.4513)
  line L3067 (-26.7444, -51.118) -> (-25.4944, -53.2831)
  line L3068 (-1.5, -51.118) -> (-2.75, -48.9529)
  line L3069 (-96.35, -47.6164) -> (-93.85, -47.6164)
  line L3070 (-88.7768, -50.5315) -> (-87.5268, -48.3664)
  line L3071 (-12.8722, -48.9529) -> (-15.3722, -48.9529)
  line L3072 (-22.9944, -48.9529) -> (-25.4944, -48.9529)
  line L3073 (-30.5435, -51.868) -> (-31.7935, -54.0331)
  line L3074 (-11.549, -54.0331) -> (-10.299, -56.1981)
  line L3075 (-26.7935, -54.0331) -> (-28.0435, -51.868)
  line L3076 (-87.5268, -48.3664) -> (-88.7768, -46.2013)
  line L3077 (-21.6713, -54.0331) -> (-20.4213, -56.1981)
  line L3078 (-78.6546, -50.5315) -> (-77.4046, -48.3664)
  line L3079 (-77.4046, -48.3664) -> (-78.6546, -46.2013)
  line L3080 (-46.9889, -45.4513) -> (-45.7389, -47.6164)
  line L3081 (-93.85, -43.2863) -> (-96.35, -43.2863)
  line L3082 (-93.85, -47.6164) -> (-92.6, -45.4513)
  line L3083 (-22.9944, -53.2831) -> (-21.7444, -51.118)
  line L3084 (-98.899, -50.5315) -> (-97.649, -48.3664)
  line L3085 (-2.75, -48.9529) -> (-5.25, -48.9529)
  line L3086 (-7.799, -56.1981) -> (-6.549, -54.0331)
  line L3087 (-26.7935, -48.3664) -> (-28.0435, -46.2013)
  line L3088 (-83.7278, -47.6164) -> (-82.4778, -45.4513)
  line L3089 (-11.6222, -51.118) -> (-12.8722, -48.9529)
  line L3090 (-7.799, -51.868) -> (-10.299, -51.868)
  line L3091 (-28.0435, -56.1981) -> (-26.7935, -54.0331)
  line L3092 (-91.2768, -50.5315) -> (-88.7768, -50.5315)
  line L3093 (-88.7768, -46.2013) -> (-91.2768, -46.2013)
  line L3094 (-82.4046, -48.3664) -> (-81.1546, -50.5315)
  line L3095 (-98.899, -46.2013) -> (-101.399, -46.2013)
  line L3096 (-33.1167, -47.6164) -> (-31.8667, -45.4513)
  line L3097 (-6.5, -51.118) -> (-5.25, -53.2831)
  line L3098 (-21.7444, -51.118) -> (-22.9944, -48.9529)
  line L3099 (-25.4944, -53.2831) -> (-22.9944, -53.2831)
  line L3100 (-81.1546, -50.5315) -> (-78.6546, -50.5315)
  line L3101 (-2.75, -53.2831) -> (-1.5, -51.118)
  line L3102 (-86.2278, -47.6164) -> (-83.7278, -47.6164)
  line L3103 (-15.3722, -53.2831) -> (-12.8722, -53.2831)
  line L3104 (-102.649, -48.3664) -> (-101.399, -50.5315)
  line L3105 (-43.2389, -48.9529) -> (-45.7389, -48.9529)
  line L3106 (-91.2768, -51.868) -> (-92.5268, -54.0331)
  line L3107 (-48.2879, -56.1981) -> (-47.0379, -54.0331)
  line L3108 (-72.3556, -51.118) -> (-73.6056, -48.9529)
  line L3109 (-5.25, -48.9529) -> (-6.5, -51.118)
  line L3110 (-41.9157, -54.0331) -> (-40.6657, -56.1981)
  line L3111 (-73.6056, -53.2831) -> (-72.3556, -51.118)
  line L3112 (-78.6546, -56.1981) -> (-77.4046, -54.0331)
  line L3113 (-68.5324, -51.868) -> (-71.0324, -51.868)
  line L3114 (-82.4778, -51.118) -> (-83.7278, -48.9529)
  line L3115 (-88.7768, -51.868) -> (-91.2768, -51.868)
  line L3116 (-77.3556, -51.118) -> (-76.1056, -53.2831)
  line L3117 (-92.5268, -54.0331) -> (-91.2768, -56.1981)
  line L3118 (-83.7278, -53.2831) -> (-82.4778, -51.118)
  line L3119 (-38.1657, -56.1981) -> (-36.9157, -54.0331)
  line L3120 (-62.1601, -54.0331) -> (-60.9101, -56.1981)
  line L3121 (-63.4833, -53.2831) -> (-62.2333, -51.118)
  line L3122 (-53.3611, -53.2831) -> (-52.1111, -51.118)
  line L3123 (-77.4046, -54.0331) -> (-78.6546, -51.868)
  line L3124 (-52.0379, -54.0331) -> (-50.7879, -56.1981)
  line L3125 (-62.2333, -51.118) -> (-63.4833, -48.9529)
  line L3126 (-36.9157, -54.0331) -> (-38.1657, -51.868)
  line L3127 (-78.6546, -51.868) -> (-81.1546, -51.868)
  line L3128 (-33.1167, -48.9529) -> (-35.6167, -48.9529)
  line L3129 (-72.2824, -54.0331) -> (-71.0324, -56.1981)
  line L3130 (-76.1056, -53.2831) -> (-73.6056, -53.2831)
  line L3131 (-91.2768, -46.2013) -> (-92.5268, -48.3664)
  line L3132 (-31.7935, -54.0331) -> (-30.5435, -56.1981)
  line L3133 (-40.6657, -56.1981) -> (-38.1657, -56.1981)
  line L3134 (-45.7389, -48.9529) -> (-46.9889, -51.118)
  line L3135 (-57.1601, -54.0331) -> (-58.4101, -51.868)
  line L3136 (-81.1546, -51.868) -> (-82.4046, -54.0331)
  line L3137 (-81.1546, -56.1981) -> (-78.6546, -56.1981)
  line L3138 (-87.4778, -51.118) -> (-86.2278, -53.2831)
  line L3139 (-58.4101, -51.868) -> (-60.9101, -51.868)
  line L3140 (-86.2278, -53.2831) -> (-83.7278, -53.2831)
  line L3141 (-45.7389, -53.2831) -> (-43.2389, -53.2831)
  line L3142 (-40.6657, -51.868) -> (-41.9157, -54.0331)
  line L3143 (-53.3611, -48.9529) -> (-55.8611, -48.9529)
  line L3144 (-43.2389, -53.2831) -> (-41.9889, -51.118)
  line L3145 (-52.1111, -51.118) -> (-53.3611, -48.9529)
  line L3146 (-91.2768, -56.1981) -> (-88.7768, -56.1981)
  line L3147 (-67.2824, -54.0331) -> (-68.5324, -51.868)
  line L3148 (-46.9889, -51.118) -> (-45.7389, -53.2831)
  line L3149 (-50.7879, -51.868) -> (-52.0379, -54.0331)
  line L3150 (-83.7278, -43.2863) -> (-86.2278, -43.2863)
  line L3151 (-67.2333, -51.118) -> (-65.9833, -53.2831)
  line L3152 (-92.5268, -48.3664) -> (-91.2768, -50.5315)
  line L3153 (-48.2879, -51.868) -> (-50.7879, -51.868)
  line L3154 (-35.6167, -48.9529) -> (-36.8667, -51.118)
  line L3155 (-76.1056, -48.9529) -> (-77.3556, -51.118)
  line L3156 (-15.3722, -48.9529) -> (-16.6222, -51.118)
  line L3157 (-82.4778, -45.4513) -> (-83.7278, -43.2863)
  line L3158 (-60.9101, -56.1981) -> (-58.4101, -56.1981)
  line L3159 (-71.0324, -56.1981) -> (-68.5324, -56.1981)
  line L3160 (-41.9889, -51.118) -> (-43.2389, -48.9529)
  line L3161 (-58.4101, -56.1981) -> (-57.1601, -54.0331)
  line L3162 (-68.5324, -56.1981) -> (-67.2824, -54.0331)
  line L3163 (-71.0324, -51.868) -> (-72.2824, -54.0331)
  line L3164 (-38.1657, -51.868) -> (-40.6657, -51.868)
  line L3165 (-47.0379, -54.0331) -> (-48.2879, -51.868)
  line L3166 (-16.6222, -51.118) -> (-15.3722, -53.2831)
  line L3167 (-97.6, -45.4513) -> (-96.35, -47.6164)
  line L3168 (-101.399, -50.5315) -> (-98.899, -50.5315)
  line L3169 (-25.4944, -58.9497) -> (-22.9944, -58.9497)
  line L3170 (-12.8722, -54.6196) -> (-15.3722, -54.6196)
  line L3171 (-6.549, -59.6997) -> (-7.799, -57.5347)
  line L3172 (-17.9213, -61.8648) -> (-16.6713, -59.6997)
  line L3173 (-38.1657, -57.5347) -> (-40.6657, -57.5347)
  line L3174 (-10.299, -61.8648) -> (-7.799, -61.8648)
  line L3175 (-46.9889, -56.7847) -> (-45.7389, -58.9497)
  line L3176 (-22.9944, -58.9497) -> (-21.7444, -56.7847)
  line L3177 (-21.7444, -56.7847) -> (-22.9944, -54.6196)
  line L3178 (-65.9833, -53.2831) -> (-63.4833, -53.2831)
  line L3179 (-12.8722, -58.9497) -> (-11.6222, -56.7847)
  line L3180 (-22.9944, -54.6196) -> (-25.4944, -54.6196)
  line L3181 (-101.399, -56.1981) -> (-98.899, -56.1981)
  line L3182 (-97.649, -54.0331) -> (-98.899, -51.868)
  line L3183 (-26.7444, -56.7847) -> (-25.4944, -58.9497)
  line L3184 (-98.899, -51.868) -> (-101.399, -51.868)
  line L3185 (-40.6657, -61.8648) -> (-38.1657, -61.8648)
  line L3186 (-15.3722, -58.9497) -> (-12.8722, -58.9497)
  line L3187 (-28.0435, -57.5347) -> (-30.5435, -57.5347)
  line L3188 (-31.7935, -59.6997) -> (-30.5435, -61.8648)
  line L3189 (-21.6713, -59.6997) -> (-20.4213, -61.8648)
  line L3190 (-15.3722, -54.6196) -> (-16.6222, -56.7847)
  line L3191 (-97.6, -51.118) -> (-96.35, -53.2831)
  line L3192 (-60.9101, -51.868) -> (-62.1601, -54.0331)
  line L3193 (-30.5435, -61.8648) -> (-28.0435, -61.8648)
  line L3194 (-10.299, -57.5347) -> (-11.549, -59.6997)
  line L3195 (-5.25, -58.9497) -> (-2.75, -58.9497)
  line L3196 (-11.549, -59.6997) -> (-10.299, -61.8648)
  line L3197 (-6.5, -56.7847) -> (-5.25, -58.9497)
  line L3198 (-33.1167, -58.9497) -> (-31.8667, -56.7847)
  line L3199 (-38.1657, -61.8648) -> (-36.9157, -59.6997)
  line L3200 (-36.9157, -59.6997) -> (-38.1657, -57.5347)
  line L3201 (-63.4833, -48.9529) -> (-65.9833, -48.9529)
  line L3202 (-31.8667, -56.7847) -> (-33.1167, -54.6196)
  line L3203 (-65.9833, -48.9529) -> (-67.2333, -51.118)
  line L3204 (-86.2278, -48.9529) -> (-87.4778, -51.118)
  line L3205 (-40.6657, -57.5347) -> (-41.9157, -59.6997)
  line L3206 (-96.35, -48.9529) -> (-97.6, -51.118)
  line L3207 (-2.75, -54.6196) -> (-5.25, -54.6196)
  line L3208 (-28.0435, -61.8648) -> (-26.7935, -59.6997)
  line L3209 (-55.8611, -48.9529) -> (-57.1111, -51.118)
  line L3210 (-16.6222, -56.7847) -> (-15.3722, -58.9497)
  line L3211 (-50.7879, -56.1981) -> (-48.2879, -56.1981)
  line L3212 (-92.6, -51.118) -> (-93.85, -48.9529)
  line L3213 (-26.7935, -59.6997) -> (-28.0435, -57.5347)
  line L3214 (-101.399, -51.868) -> (-102.649, -54.0331)
  line L3215 (-35.6167, -58.9497) -> (-33.1167, -58.9497)
  line L3216 (-17.9213, -57.5347) -> (-20.4213, -57.5347)
  line L3217 (-16.6713, -59.6997) -> (-17.9213, -57.5347)
  line L3218 (-87.5268, -54.0331) -> (-88.7768, -51.868)
  line L3219 (-93.85, -53.2831) -> (-92.6, -51.118)
  line L3220 (-33.1167, -54.6196) -> (-35.6167, -54.6196)
  line L3221 (-7.799, -57.5347) -> (-10.299, -57.5347)
  line L3222 (-30.5435, -57.5347) -> (-31.7935, -59.6997)
  line L3223 (-36.8667, -56.7847) -> (-35.6167, -58.9497)
  line L3224 (-20.4213, -61.8648) -> (-17.9213, -61.8648)
  line L3225 (-20.4213, -57.5347) -> (-21.6713, -59.6997)
  line L3226 (-7.799, -61.8648) -> (-6.549, -59.6997)
  line L3227 (-55.8611, -53.2831) -> (-53.3611, -53.2831)
  line L3228 (-5.25, -54.6196) -> (-6.5, -56.7847)
  line L3229 (-83.7278, -48.9529) -> (-86.2278, -48.9529)
  line L3230 (-73.6056, -48.9529) -> (-76.1056, -48.9529)
  line L3231 (-57.1111, -51.118) -> (-55.8611, -53.2831)
  line L3232 (-82.4046, -54.0331) -> (-81.1546, -56.1981)
  line L3233 (-62.1601, -59.6997) -> (-60.9101, -61.8648)
  line L3234 (-73.6056, -54.6196) -> (-76.1056, -54.6196)
  line L3235 (-98.899, -56.1981) -> (-97.649, -54.0331)
  line L3236 (-73.6056, -58.9497) -> (-72.3556, -56.7847)
  line L3237 (-52.1111, -56.7847) -> (-53.3611, -54.6196)
  line L3238 (-2.75, -58.9497) -> (-1.5, -56.7847)
  line L3239 (-87.5268, -59.6997) -> (-88.7768, -57.5347)
  line L3240 (-97.6, -56.7847) -> (-96.35, -58.9497)
  line L3241 (-71.0324, -61.8648) -> (-68.5324, -61.8648)
  line L3242 (-76.1056, -58.9497) -> (-73.6056, -58.9497)
  line L3243 (-93.85, -54.6196) -> (-96.35, -54.6196)
  line L3244 (-47.0379, -59.6997) -> (-48.2879, -57.5347)
  line L3245 (-96.35, -53.2831) -> (-93.85, -53.2831)
  line L3246 (-57.1601, -59.6997) -> (-58.4101, -57.5347)
  line L3247 (-50.7879, -57.5347) -> (-52.0379, -59.6997)
  line L3248 (-1.5, -56.7847) -> (-2.75, -54.6196)
  line L3249 (-53.3611, -54.6196) -> (-55.8611, -54.6196)
  line L3250 (-11.6222, -56.7847) -> (-12.8722, -54.6196)
  line L3251 (-55.8611, -54.6196) -> (-57.1111, -56.7847)
  line L3252 (-87.4778, -56.7847) -> (-86.2278, -58.9497)
  line L3253 (-50.7879, -61.8648) -> (-48.2879, -61.8648)
  line L3254 (-41.9889, -56.7847) -> (-43.2389, -54.6196)
  line L3255 (-41.9157, -59.6997) -> (-40.6657, -61.8648)
  line L3256 (-63.4833, -54.6196) -> (-65.9833, -54.6196)
  line L3257 (-93.85, -48.9529) -> (-96.35, -48.9529)
  line L3258 (-48.2879, -57.5347) -> (-50.7879, -57.5347)
  line L3259 (-83.7278, -58.9497) -> (-82.4778, -56.7847)
  line L3260 (-88.7768, -56.1981) -> (-87.5268, -54.0331)
  line L3261 (-43.2389, -54.6196) -> (-45.7389, -54.6196)
  line L3262 (-72.2824, -59.6997) -> (-71.0324, -61.8648)
  line L3263 (-83.7278, -54.6196) -> (-86.2278, -54.6196)
  line L3264 (-55.8611, -58.9497) -> (-53.3611, -58.9497)
  line L3265 (-92.5268, -59.6997) -> (-91.2768, -61.8648)
  line L3266 (-65.9833, -58.9497) -> (-63.4833, -58.9497)
  line L3267 (-67.2824, -59.6997) -> (-68.5324, -57.5347)
  line L3268 (-71.0324, -57.5347) -> (-72.2824, -59.6997)
  line L3269 (-91.2768, -57.5347) -> (-92.5268, -59.6997)
  line L3270 (-93.85, -58.9497) -> (-92.6, -56.7847)
  line L3271 (-68.5324, -61.8648) -> (-67.2824, -59.6997)
  line L3272 (-45.7389, -58.9497) -> (-43.2389, -58.9497)
  line L3273 (-88.7768, -57.5347) -> (-91.2768, -57.5347)
  line L3274 (-86.2278, -54.6196) -> (-87.4778, -56.7847)
  line L3275 (-78.6546, -57.5347) -> (-81.1546, -57.5347)
  line L3276 (-52.0379, -59.6997) -> (-50.7879, -61.8648)
  line L3277 (-88.7768, -61.8648) -> (-87.5268, -59.6997)
  line L3278 (-65.9833, -54.6196) -> (-67.2333, -56.7847)
  line L3279 (-77.4046, -59.6997) -> (-78.6546, -57.5347)
  line L3280 (-72.3556, -56.7847) -> (-73.6056, -54.6196)
  line L3281 (-43.2389, -58.9497) -> (-41.9889, -56.7847)
  line L3282 (-82.4046, -59.6997) -> (-81.1546, -61.8648)
  line L3283 (-25.4944, -54.6196) -> (-26.7444, -56.7847)
  line L3284 (-62.2333, -56.7847) -> (-63.4833, -54.6196)
  line L3285 (-60.9101, -57.5347) -> (-62.1601, -59.6997)
  line L3286 (-102.649, -54.0331) -> (-101.399, -56.1981)
  line L3287 (-77.3556, -56.7847) -> (-76.1056, -58.9497)
  line L3288 (-81.1546, -61.8648) -> (-78.6546, -61.8648)
  line L3289 (-82.4778, -56.7847) -> (-83.7278, -54.6196)
  line L3290 (-86.2278, -58.9497) -> (-83.7278, -58.9497)
  line L3291 (-67.2333, -56.7847) -> (-65.9833, -58.9497)
  line L3292 (-76.1056, -54.6196) -> (-77.3556, -56.7847)
  line L3293 (-53.3611, -58.9497) -> (-52.1111, -56.7847)
  line L3294 (-81.1546, -57.5347) -> (-82.4046, -59.6997)
  line L3295 (-45.7389, -54.6196) -> (-46.9889, -56.7847)
  line L3296 (-35.6167, -54.6196) -> (-36.8667, -56.7847)
  line L3297 (-16.6222, -62.4513) -> (-15.3722, -64.6164)
  line L3298 (-102.649, -59.6997) -> (-101.399, -61.8648)
  line L3299 (-36.9157, -65.3664) -> (-38.1657, -63.2013)
  line L3300 (-35.6167, -64.6164) -> (-33.1167, -64.6164)
  line L3301 (-31.8667, -62.4513) -> (-33.1167, -60.2863)
  line L3302 (-16.6713, -65.3664) -> (-17.9213, -63.2013)